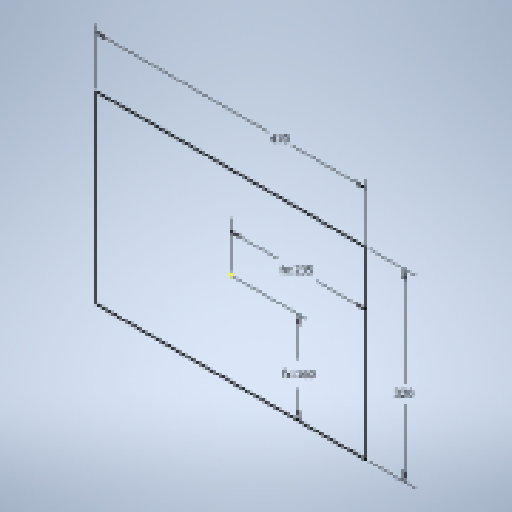
# Autodesk Inventor part: Base
Saved by Autodesk Inventor 2023.1 (Build 271208000, 208)
## iProperties
Created: 2022-11-11
Part Number: Base
Material: MDF Medium Density Fiberboard
Document SubType Name: Modeling
Designer: Daniel Peña
Density: 0.8 g/cm^3
Appearance: Chestnut
Author: Daniel Peña
Autodesk Inventor part; units mm, degrees
ref_plane "YZ Plane" through (0, 0, 0) normal (1, 0, 0) x (0, 1, 0)
ref_plane "XZ Plane" through (0, 0, 0) normal (0, 1, 0) x (-1, 0, 0)
ref_plane "XY Plane" through (0, 0, 0) normal (0, 0, 1) x (1, 0, 0)
sketch "Sketch1" plane through (0, 0, 0) normal (0, 0, 1) x (1, 0, 0)
  line L0 (-235, 160) -> (235, 160)
  line L1 (235, 160) -> (235, -160)
  line L2 (235, -160) -> (-235, -160)
  line L3 (-235, -160) -> (-235, 160)
  point P0 (0, 0)
  dimension "d0" = 470
  dimension "d1" = 320
  dimension "d2" = 160
  dimension "d3" = 235
  constraints: 8 end point, 2 parallel, 1 horizontal, 1 perpendicular
  measures "d0" distance of L0.start L0.end
  measures "d1" distance of L0.end L1.end
  measures "d2" distance from line of L2 point (0, 0)
  measures "d3" distance from line of point (0, 0) L1
extrude "Extrusion1" add sketch "Sketch1" along normal blind 3
sketch "Sketch2" plane through (0, 0, 3) normal (0, 0, 1) x (1, 0, 0)
  line L0 (235, 160) -> (-235, 160) construction
  line L1 (0, 160) -> (0, -160) construction
  line L2 (-235, -160) -> (235, -160) construction
  line L3 (-235, 160) -> (-235, -160) construction
  line L4 (-235, 0) -> (235, 0) construction
  line L5 (235, -160) -> (235, 160) construction
  point P0 (0, 0)
  point P1 (-220, 145)
  point P2 (-220, -145)
  point P3 (220, -145)
  point P4 (220, 145)
  dimension "d6" = 15
  dimension "d7" = 15
  constraints: 4 end point, 4 midpoint, 3 symmetric about line
  measures "d6" distance from line of L2 point (-220, -145)
  measures "d7" distance from line of L3 point (-220, -145)
hole "Hole1" at (-220, 145, 3) at (-220, -145, 3) at (220, -145, 3) at (220, 145, 3) direction (0, 0, -1) diameter 5.1 end through all
equation "\"d2\" = 0.5 * d1"
equation "\"d3\" = 0.5 * d0"
body "Solid1"
